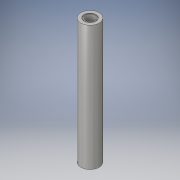
# Autodesk Inventor part: LED holder Thing
Saved by Autodesk Inventor 2016 (Build 200138000, 138)
## iProperties
Created: 2017-09-26
Part Number: LED holder Thing
Material: Generic
Document SubType Name: Modeling
Designer: Student
Density: 1 g/cm^3
Appearance: Default
Author: Student
Autodesk Inventor part; units mm, degrees
ref_plane "YZ Plane" through (0, 0, 0) normal (1, 0, 0) x (0, 1, 0)
ref_plane "XZ Plane" through (0, 0, 0) normal (0, 1, 0) x (-1, 0, 0)
ref_plane "XY Plane" through (0, 0, 0) normal (0, 0, 1) x (1, 0, 0)
sketch "Sketch1" plane through (0, 0, 0) normal (0, 1, 0) x (-1, 0, 0)
  circle A0 centre (0, 0) radius 22.1996
  dimension "d0" = 44.3992
  constraints: 1 centre point, 1 coincident
  measures "d0" diameter of A0
extrude "Extrusion1" add sketch "Sketch1" along normal blind 305.1302
sketch "Sketch2" plane through (0, 305.1302, 0) normal (0, 1, 0) x (1, 0, 0)
  circle A0 centre (0, 0) radius 14.4526
  circle A1 centre (0, 0) radius 12.6365
  dimension "d3" = 28.9052
  dimension "d4" = 25.273
  constraints: 2 centre point, 2 coincident
  measures "d3" diameter of A0
  measures "d4" diameter of A1
extrude "Extrusion2" cut sketch "Sketch2" against normal blind 1.8034
sketch "Sketch3" plane through (0, 305.1302, 0) normal (0, 1, 0) x (1, 0, 0)
  circle A0 centre (0, 0) radius 10.9441
  circle A1 centre (0, 0) radius 12.6365 projected
  dimension "d7" = 1.6924
  constraints: 1 centre point, 1 coincident
  measures "d7" radial gap between concentric circles of A1 A0
extrude "Extrusion3" cut sketch "Sketch3" against normal blind 14.6558 draft -17 contours A0
sketch "Sketch5" plane through (0, 290.4744, 0) normal (0, 1, 0) x (1, 0, 0)
  circle A0 centre (0, 0) radius 6.4634
  constraints: 1 centre point, 1 coincident
extrude "Extrusion4" cut sketch "Sketch5" against normal blind 355.6
sketch "Sketch6" plane through (0, 0, 0) normal (0, -1, 0) x (1, 0, 0)
  circle A0 centre (0, 0) radius 19.05
  circle A1 centre (0, 0) radius 22.1996
  dimension "d13" = 38.1
  dimension "d14" = 44.3992
  constraints: 2 centre point, 2 coincident
  measures "d13" diameter of A0
  measures "d14" diameter of A1
extrude "Extrusion5" cut sketch "Sketch6" against normal blind 290.449 contours A0
body "Solid1"
